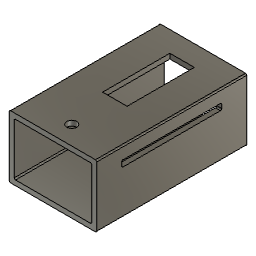
heating_pad_electronics_box (Autodesk Fusion 360 design; units mm, degrees)
Autodesk Fusion 360 part; units mm, degrees
sketch "Sketch1" plane through (0, 0, 0) normal (0, 1, 0) x (1, 0, 0)
  line L0 (-65, 0) -> (50, 0) construction
  line L1 (-34, -25) -> (34, -25)
  line L2 (35, -24) -> (35, 24)
  line L3 (34, 25) -> (-34, 25)
  line L4 (-35, 24) -> (-35, -24)
  line L5 (-35, 25) -> (35, -25) construction
  line L6 (-35, -25) -> (35, 25) construction
  arc A0 (-35, -24) -> (-34, -25) centre (-34, -24) ccw
  arc A1 (34, -25) -> (35, -24) centre (34, -24) ccw
  arc A2 (35, 24) -> (34, 25) centre (34, 24) ccw
  arc A3 (-34, 25) -> (-35, 24) centre (-34, 24) ccw
  point P0 (-32.7786, 20)
  point P1 (32.2214, 20)
  point P2 (-32.7786, -20)
  dimension "d7" = 70
  dimension "d8" = 50
  dimension "d9" = 1
  dimension "d10" = 1
  constraint horizontal L1
  constraint vertical L2
  constraint horizontal L3
  constraint vertical L4
  constraint coincident origin L5
  constraint midpoint L5 origin
  constraint coincident L6.start L4
  constraint coincident L6.start L1
  constraint tangent L4 A0
  constraint tangent L1 A0
  constraint coincident L5.end L2
  constraint coincident L5.end L1
  constraint tangent L2 A1
  constraint tangent L1 A1
  constraint equal A0 A1
  constraint coincident L6.end L2
  constraint coincident L6.end L3
  constraint tangent L2 A2
  constraint tangent L3 A2
  constraint equal A0 A2
  constraint coincident L5.start L3
  constraint coincident L5.start L4
  constraint tangent L3 A3
  constraint tangent L4 A3
  measures "d7" distance of L6.start L5.end
  measures "d8" distance of L6.start L5.start
  measures "d9" radius of A0
  measures "d10" radius of A3
extrude "Extrude1" add sketch "Sketch1" along normal mid plane 120
sketch "Sketch2" plane through (0, -60, 0) normal (0, -1, 0) x (1, 0, 0)
  arc A0 (-35, -24) -> (-34, -25) centre (-34, -24) ccw
  line L0 (-34, -25) -> (34, -25)
  arc A1 (34, -25) -> (35, -24) centre (34, -24) ccw
  line L1 (35, -24) -> (35, 24)
  arc A2 (35, 24) -> (34, 25) centre (34, 24) ccw
  line L2 (34, 25) -> (-34, 25)
  arc A3 (-34, 25) -> (-35, 24) centre (-34, 24) ccw
  line L3 (-35, 24) -> (-35, -24)
  line L4 (-29.9936, -20.9993) -> (29.9936, -20.9993)
  line L5 (30.9936, -19.9993) -> (30.9936, 19.9993)
  line L6 (29.9936, 20.9993) -> (-29.9936, 20.9993)
  line L7 (-30.9936, 19.9993) -> (-30.9936, -19.9993)
  arc A4 (-29.9936, 20.9993) -> (-30.9936, 19.9993) centre (-29.9936, 19.9993) ccw
  arc A5 (30.9936, 19.9993) -> (29.9936, 20.9993) centre (29.9936, 19.9993) ccw
  arc A6 (29.9936, -20.9993) -> (30.9936, -19.9993) centre (29.9936, -19.9993) ccw
  arc A7 (-30.9936, -19.9993) -> (-29.9936, -20.9993) centre (-29.9936, -19.9993) ccw
  line L8 (-45, 0) -> (50, 0) construction
  line L9 (0, 30) -> (0, -30) construction
  dimension "d11" = 1
  constraint horizontal L4
  constraint vertical L5
  constraint horizontal L6
  constraint vertical L7
  constraint tangent L7 A4
  constraint tangent L6 A4
  constraint tangent L5 A5
  constraint tangent L6 A5
  constraint equal A4 A5
  constraint tangent L5 A6
  constraint tangent L4 A6
  constraint equal A4 A6
  constraint tangent L4 A7
  constraint tangent L7 A7
  constraint equal A4 A7
  constraint perpendicular L5 L8
  constraint perpendicular L0 L9
  constraint symmetric L4 L6 L8
  measures "d11" radius of A4
extrude "Extrude2" cut sketch "Sketch2" against normal blind 120 contours L4 L5 L6 L7 A4 A5 A6 A7
sketch "Sketch3" plane through (0, 0, 25) normal (0, 0, 1) x (-1, 0, 0)
  line L0 (-34, 60) -> (-34, -60)
  line L1 (-34, -60) -> (34, -60)
  line L2 (34, -60) -> (34, 60)
  line L3 (34, 60) -> (-34, 60)
  circle A0 centre (0, 45) radius 4
  line L4 (10, 10.3084) -> (-9.5736, 10.3084)
  line L5 (-9.5736, 10.3084) -> (-9.5736, -43.5288)
  line L6 (-9.5736, -43.5288) -> (10, -43.5288)
  line L7 (10, -43.5288) -> (10, 10.3084)
  dimension "d14" = 8
  constraint horizontal L4
  constraint vertical L5
  constraint horizontal L6
  constraint vertical L7
  measures "d14" diameter of A0
extrude "Extrude3" cut sketch "Sketch3" against normal blind 5 contours A0 | L4 L5 L6 L7
sketch "Sketch4" plane through (35, 0, 0) normal (1, 0, 0) x (0, 1, 0)
  line L0 (-60, -24) -> (60, -24)
  line L1 (60, -24) -> (60, 24)
  line L2 (60, 24) -> (-60, 24)
  line L3 (-60, 24) -> (-60, -24)
  line L4 (-39, 15) -> (39, 15)
  line L5 (40, 14) -> (40, 11)
  line L6 (39, 10) -> (-39, 10)
  line L7 (-40, 11) -> (-40, 14)
  arc A0 (-39, 15) -> (-40, 14) centre (-39, 14) ccw
  arc A1 (40, 14) -> (39, 15) centre (39, 14) ccw
  arc A2 (39, 10) -> (40, 11) centre (39, 11) ccw
  arc A3 (-40, 11) -> (-39, 10) centre (-39, 11) ccw
  dimension "d17" = 1
  constraint horizontal L4
  constraint vertical L5
  constraint horizontal L6
  constraint vertical L7
  constraint tangent L4 A0
  constraint tangent L7 A0
  constraint tangent L5 A1
  constraint tangent L4 A1
  constraint equal A0 A1
  constraint tangent L6 A2
  constraint tangent L5 A2
  constraint equal A0 A2
  constraint tangent L6 A3
  constraint tangent L7 A3
  constraint equal A0 A3
  measures "d17" radius of A0
extrude "Extrude4" cut sketch "Sketch4" against normal blind 5 contours L4 L5 L6 L7 A0 A1 A2 A3
